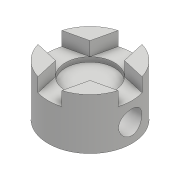
# Autodesk Inventor part: embrague_2_1
Saved by Autodesk Inventor 2018 (Build 220112000, 112)
## iProperties
Created: 2018-08-07
Part Number: embrague_2_1
Material: Generic
Document SubType Name: Sheet Metal
Designer: Bardo91
Density: 1 g/cm^3
Sheet Metal Rule: Default_mm
Appearance: Default
Author: Bardo91
Autodesk Inventor part; units mm, degrees
ref_plane "YZ Plane" through (0, 0, 0) normal (1, 0, 0) x (0, 1, 0)
ref_plane "XZ Plane" through (0, 0, 0) normal (0, 1, 0) x (-1, 0, 0)
ref_plane "XY Plane" through (0, 0, 0) normal (0, 0, 1) x (1, 0, 0)
sketch "Sketch8" plane through (0, 0, 0) normal (0, 0, 1) x (1, 0, 0)
  circle A0 centre (0, 0) radius 9
  dimension "d50" = 18
  constraints: 1 centre point
  measures "d50" diameter of A0
extrude "Extrusion8" add sketch "Sketch8" along normal blind 8
sketch "Sketch12" plane through (0, 0, 0) normal (1, 0, 0) x (0, 1, 0)
  line L0 (9, 8) -> (-9, 8) projected
  line L1 (0, 8) -> (0, 0)
  circle A0 centre (0, 4) radius 2.5
  dimension "d63" = 5
  constraints: 2 end point, 2 midpoint, 1 centre point, 1 vertical
  measures "d63" diameter of A0
extrude "Extrusion11" cut sketch "Sketch12" along normal through all both and the other way through all
sketch "Sketch16" plane through (0, 0, 8) normal (0, 0, 1) x (1, 0, 0)
  circle A0 centre (0, 0) radius 9
  constraints: 1 centre point, 1 coincident
extrude "Extrusion13" add sketch "Sketch16" along normal blind 3
sketch "Sketch15" plane through (0, 0, 8) normal (0, 0, 1) x (1, 0, 0)
  arc A0 (-3.7123, -3.7123) -> (-5.25, 0) centre (0, 0) ccw
  line L0 (0, 0) -> (-9, 0)
  circle A1 centre (0, 0) radius 9 projected
  line L1 (-9, 0) -> (-9, 2.5)
  line L2 (0, 0) -> (-3.7123, 3.7123)
  line L3 (0, 0) -> (5.25, 0) construction
  line L4 (-3.7123, 3.7123) -> (-9, 2.5)
  line L5 (-9, 0) -> (-9, -2.5)
  line L6 (-3.7123, -3.7123) -> (-9, -2.5)
  line L7 (0, 0) -> (0, 9)
  line L8 (0, 9) -> (-2.5, 9)
  line L9 (-2.5, 9) -> (-3.7123, 3.7123)
  line L10 (0, 9) -> (2.5, 9)
  line L11 (2.5, 9) -> (3.7123, 3.7123)
  line L12 (0, 0) -> (9, 0)
  line L13 (9, 0) -> (9, 2.5)
  line L14 (9, 2.5) -> (3.7123, 3.7123)
  line L15 (9, 0) -> (9, -2.5)
  line L16 (9, -2.5) -> (3.7123, -3.7123)
  line L17 (0, -9) -> (-2.5, -9)
  line L18 (-2.5, -9) -> (-3.7123, -3.7123)
  line L19 (0, -9) -> (2.5, -9)
  line L20 (2.5, -9) -> (3.7123, -3.7123)
  dimension "d68" = 10.5
  dimension "d69" = 9
  dimension "d70" = 2.5
  dimension "d71" = 135
  dimension "d72" = 9
  dimension "d73" = 2.5
  dimension "d74" = 2.5
  dimension "d75" = 2.5
  dimension "d76" = 2.5
  dimension "d77" = 2.5
  dimension "d78" = 2.5
  constraints: 42 end point, 7 point on circle, 6 point on line, 4 perpendicular, 3 tangent, 2 horizontal, 2 symmetric about line, 1 centre point, 1 coincident, 1 equal length, 1 vertical
  measures "d68" diameter of A0
  measures "d69" distance of L0.start L0.end
  measures "d70" distance of L0.end L1.end
  measures "d71" angle of L3 L2
  measures "d72" distance of L2.start L7.end
  measures "d73" distance of L7.end L8.end
  measures "d74" distance of L7.end L10.end
  measures "d75" distance of L12.end L13.end
  measures "d76" distance of L12.end L15.end
  measures "d77" distance of L17.start L17.end
  measures "d78" distance of L17.start L19.end
extrude "Extrusion14" cut sketch "Sketch15" along normal blind 3 contours L6 A1 L0 L12 A0 | A0 L20 A1 L18 | A0 L12 A1 L16 | L6 L5 A1 | A1 L17 L18 | L12 L7 A0 | A0 L14 A1 L12 | A1 L15 L16 | L20 L19 A1 | A1 L4 A0 L0 | L1 L4 A1 | A0 L7 A1 L11 | L0 A0 L2 | L2 A0 L7 | A1 L14 L13 | A0 L9 A1 L7 | A1 L10 L11 | L9 L8 A1
sketch "Sketch17" plane through (0, 0, 8) normal (0, 0, 1) x (1, 0, 0)
  line L0 (8.6201, 2.5871) -> (3.7123, 3.7123) projected
  circle A0 centre (0, 0) radius 5.25
  constraints: 1 coincident, 3 other
extrude "Extrusion15" cut sketch "Sketch17" against normal blind 1
equation "\"BendRadius\" = Thickness"
equation "\"BendReliefWidth\" = Thickness"
equation "\"BendReliefDepth\" = 0.5 * Thickness"
equation "\"CornerReliefSize\" = 4 * Thickness"
equation "\"MinimumRemnant\" = 2 * Thickness"
equation "\"TransitionRadius\" = BendRadius"
equation "\"JacobiRadiusSize\" = BendRadius"
equation "\"GapSize\" = Thickness"
equation "\"Thickness\" = 0.5"
body "Solid2"
